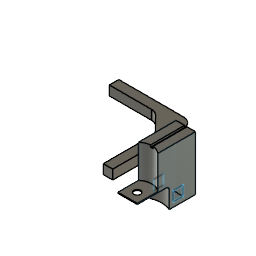
motor_holder_2 (Autodesk Fusion 360 design; units mm, degrees)
part number: 2025-11-13-17-57-27-418
part number: 2025-11-14-11-12-25-876
part number: 2025-11-14-11-12-42-976
Autodesk Fusion 360 part; units mm, degrees
sketch "Sketch1" plane through (0, 0, 0) normal (0, 0, 1) x (1, 0, 0)
  line L0 (0, 0) -> (100, 0)
  line L1 (100, 0) -> (100, 30)
  line L2 (100, 30) -> (0, 30)
  line L3 (0, 30) -> (0, 0)
  line L4 (20, 30) -> (80, 30)
  line L5 (80, 30) -> (80, 0)
  line L6 (80, 0) -> (20, 0)
  line L7 (20, 0) -> (20, 30)
  dimension "d1" = 100
  dimension "d2" = 30
  dimension "d3" = 60
  constraint horizontal L0
  constraint vertical L1
  constraint horizontal L2
  constraint vertical L3
  constraint coincident L0.start L3.end
  constraint horizontal L4
  constraint vertical L5
  constraint horizontal L6
  constraint vertical L7
  constraint coincident L0 L5.end
  constraint coincident L2 L4.start
  constraint midpoint L2 L4
  measures "d1" distance of L0.start L0.end
  measures "d2" distance of L0.start L2.end
  measures "d3" distance of L5 L7
extrude "Extrude2" add sketch "Sketch1" along normal blind 56 contours L0 L2 L3 L7 makes body 1
sketch "Sketch2" plane through (0, 0, 0) normal (0, -1, 0) x (1, 0, 0)
  line L0 (0, 0) -> (20, 0)
  line L1 (20, 0) -> (20, 56)
  line L2 (20, 56) -> (0, 56)
  line L3 (0, 56) -> (0, 0)
  line L4 (0, 56) -> (20, 56)
  line L5 (20, 56) -> (20, 21)
  line L6 (20, 21) -> (0, 21)
  line L7 (0, 21) -> (0, 56)
  line L8 (80, 60) -> (100, 60)
  line L9 (100, 60) -> (100, 30)
  line L10 (100, 30) -> (80, 30)
  line L11 (80, 30) -> (80, 60)
  dimension "d8" = 35
  dimension "d45" = 20
  constraint horizontal L4
  constraint vertical L5
  constraint horizontal L6
  constraint vertical L7
  constraint coincident L2.end L3.start
  constraint horizontal L8
  constraint vertical L9
  constraint horizontal L10
  constraint vertical L11
  measures "d8" distance of L2.end L6.end
  measures "d45" distance of L5 L7
extrude "Extrude3" add sketch "Sketch2" along normal blind 30 contours L1 L2 L3 L4 L5 L6 L7 bodies 1
sketch "Sketch3" plane through (0, 0, 21) normal (0, 0, -1) x (1, 0, 0)
  line L0 (20, 0) -> (20, 30)
  line L1 (20, 30) -> (0, 30)
  line L2 (0, 30) -> (0, 0)
  circle A0 centre (10, 20) radius 3.5
  line L3 (0, 0) -> (20, 0)
  dimension "d11" = 7
  dimension "d13" = 10
  dimension "d15" = 10
  measures "d11" diameter of A0
  measures "d13" distance of L1 A0.centre
  measures "d15" distance of L2 A0.centre
sketch "Sketch4" plane through (0, 0, 56) normal (0, 0, 1) x (-1, 0, 0)
  line L0 (-20, 30) -> (-20, -30)
  line L1 (-20, -30) -> (0, -30)
  line L2 (0, -30) -> (0, 30)
  line L3 (0, 30) -> (-20, 30)
  circle A0 centre (-10, 20) radius 15
  circle A1 centre (-90, 20) radius 15
  dimension "d17" = 30
  dimension "d18" = 30
  measures "d17" diameter of A0
  measures "d18" diameter of A1
extrude "Extrude4" cut sketch "Sketch4" against normal blind 34 contours L0 L2 L3 A0 picked at (-10, 21.6667) bodies 1
extrude "Extrude5" cut sketch "Sketch3" against normal blind 2 contours A0 bodies 1
sketch "Sketch6" plane through (0, 0, 21) normal (0, 0, -1) x (1, 0, 0)
  circle A0 centre (10, 20) radius 20
  circle A1 centre (10, 20) radius 25
  circle A2 centre (10, 20) radius 3.5
  line L0 (20, 30) -> (20, 8.8197)
  arc A3 (0, 8.8197) -> (20, 8.8197) centre (10, 20) ccw
  line L1 (0, 8.8197) -> (0, 30)
  line L2 (0, 30) -> (20, 30)
  circle A4 centre (10, 20) radius 3.5
  line L3 (0, 0) -> (20, 0)
  line L4 (20, 0) -> (20, 30)
  line L5 (20, 30) -> (0, 30)
  line L6 (0, 30) -> (0, 0)
  dimension "d27" = 40
  dimension "d28" = 5
  measures "d27" diameter of A0
extrude "Extrude6" cut sketch "Sketch6" along normal blind 25 contours A0 L3 L6 | A0 L3 L4 | A1 bodies 1
fillet "Fillet2" radius 3 1 edges at (10, 5, 21) on bodies 1
sketch "Sketch7" plane through (0, 0, 56) normal (0, 0, 1) x (-1, 0, 0)
  line L0 (-20, 8.8197) -> (-20, -30)
  line L1 (-20, -30) -> (0, -30)
  line L2 (0, -30) -> (0, 8.8197)
  line L3 (-8.75, 5.0522) -> (-11.25, 5.0522)
  line L4 (-11.25, 5.0522) -> (-11.25, -30)
  line L5 (-11.25, -30) -> (-8.75, -30)
  line L6 (-8.75, -30) -> (-8.75, 5.0522)
  line L7 (0, 5.0522) -> (-20, 5.0522) construction
  arc A0 (-20, 8.8197) -> (0, 8.8197) centre (-10, 20) ccw
  dimension "d33" = 2.5
  constraint horizontal L3
  constraint vertical L4
  constraint horizontal L5
  constraint vertical L6
  constraint coincident L1 L4.end
  constraint coincident L2 L7.start
  constraint coincident L0 L7.end
  constraint perpendicular L0 L7
  constraint midpoint L3 L7
  measures "d33" distance of L4 L6
sketch "Sketch8" plane through (0, 0, 0) normal (-1, 0, 0) x (0, -1, 0)
  line L0 (-2.9129, 0) -> (-2.9129, 18)
  spline S0 degree 3 poles (0.4041, 21) (-0.0235, 21) (-0.5283, 20.9083) (-1.2987, 20.607) (-1.7061, 20.3539) (-2.269, 19.8209) (-2.5307, 19.454) (-2.8238, 18.7805) (-2.9129, 18.359) (-2.9129, 18) knots 1.421755 1.421755 1.421755 1.421755 1.550024 1.550024 1.669923 1.669923 1.782589 1.782589 1.890287 1.890287 1.890287 1.890287
  line L1 (0.4041, 21) -> (30, 21)
  line L2 (30, 21) -> (30, 22)
  line L3 (30, 22) -> (8.8197, 22)
  line L4 (8.8197, 22) -> (8.8197, 56)
  line L5 (8.8197, 56) -> (-30, 56)
  line L6 (-30, 56) -> (-30, 0)
  line L7 (-30, 0) -> (-2.9129, 0)
  line L8 (-17, 15) -> (-7, 15)
  line L9 (-7, 15) -> (-7, 5)
  line L10 (-7, 5) -> (-17, 5)
  line L11 (-17, 5) -> (-17, 15)
  dimension "d37" = 10
  dimension "d38" = 5
  constraint horizontal L8
  constraint vertical L9
  constraint horizontal L10
  constraint vertical L11
  measures "d37" distance of L8.start L10.end
  measures "d38" distance of L7 L10
extrude "Extrude7" cut sketch "Sketch8" against normal blind 9 contours L8 L9 L10 L11 bodies 1
sketch "Sketch9" plane through (20, 0, 0) normal (1, 0, 0) x (0, 1, 0)
  line L0 (2.9129, 0) -> (30, 0)
  line L1 (30, 0) -> (30, 56)
  line L2 (30, 56) -> (-8.8197, 56)
  line L3 (-8.8197, 56) -> (-8.8197, 22)
  line L4 (-8.8197, 22) -> (-30, 22)
  line L5 (-30, 22) -> (-30, 21)
  line L6 (-30, 21) -> (-0.4041, 21)
  spline S0 degree 3 poles (2.9129, 18) (2.9129, 18.359) (2.8238, 18.7805) (2.5307, 19.454) (2.269, 19.8209) (1.7061, 20.3539) (1.2987, 20.607) (0.5283, 20.9083) (0.0235, 21) (-0.4041, 21) knots 0 0 0 0 0.107698 0.107698 0.220364 0.220364 0.340263 0.340263 0.468532 0.468532 0.468532 0.468532
  line L7 (2.9129, 18) -> (2.9129, 0)
  line L8 (7, 15) -> (17, 15)
  line L9 (17, 15) -> (17, 5)
  line L10 (17, 5) -> (7, 5)
  line L11 (7, 5) -> (7, 15)
  constraint horizontal L8
  constraint vertical L9
  constraint horizontal L10
  constraint vertical L11
extrude "Extrude8" cut sketch "Sketch9" against normal blind 9 contours L8 L9 L10 L11 bodies 1
extrude "Extrude9" cut sketch "Sketch7" against normal blind 2 contours L1 L4 L5 L6 A0 bodies 1
sketch "Sketch14" plane through (0, 0, 0) normal (0, 1, 0) x (1, 0, 0)
  line L0 (-45, -10) -> (-35.2, -10)
  line L1 (-35.2, -10) -> (-35.2, -0.2)
  line L2 (-35.2, -0.2) -> (-45, -0.2)
  line L3 (-45, -0.2) -> (-45, -10)
  dimension "d69" = 9.8
  dimension "d70" = 9.8
  constraint horizontal L0
  constraint vertical L1
  constraint horizontal L2
  constraint vertical L3
  measures "d69" distance of L0.start L0.end
  measures "d70" distance of L0.start L2.end
extrude "Extrude15" add sketch "Sketch14" along normal blind 83 separate body makes body 2
sketch "Sketch15" plane through (-45, 0, 0) normal (-1, 0, 0) x (0, -1, 0)
  line L0 (0, 0.2) -> (0, 10)
  line L1 (0, 10) -> (-83, 10)
  line L2 (-83, 10) -> (-83, 0.2)
  line L3 (-83, 0.2) -> (0, 0.2)
  line L4 (-83, 10) -> (-73.2, 10)
  line L5 (-73.2, 10) -> (-73.2, 0.2)
  line L6 (-73.2, 0.2) -> (-83, 0.2)
  line L7 (-83, 0.2) -> (-83, 10)
  dimension "d60" = 9.8
  dimension "d72" = 9.8
  constraint horizontal L4
  constraint vertical L5
  constraint horizontal L6
  constraint vertical L7
  constraint coincident L1.end L2.start
  measures "d60" distance of L1.end L4.end
  measures "d72" distance of L4 L6
extrude "Extrude16" add sketch "Sketch15" along normal blind 67 contours L1 L2 L3 L4 L5 L6 L7 bodies 2
copy_body "Body->Comp1" bodies 2 removing the originals makes body 3 in component "dubel"
copy_body "Body->Comp2" bodies 1 removing the originals makes body 4 in component "motor_holder"
sketch "Sketch16" plane through (0, 0, 10) normal (0, 0, 1) x (-1, 0, 0)
  line L0 (45, 0) -> (35.2, 0)
  line L1 (35.2, 0) -> (35.2, -83)
  line L2 (35.2, -83) -> (112, -83)
  line L3 (112, -83) -> (112, -73.2)
  line L4 (112, -73.2) -> (45, -73.2)
  line L5 (45, -73.2) -> (45, 0)
  line L6 (64.3141, -73.2) -> (45, -73.2)
  line L7 (45, -53.5452) -> (64.3141, -73.2)
  constraint coincident L4 L6.start
  constraint coincident L4.end L5.start
  constraint coincident L5 L7.start
extrude "Extrude1" add sketch "Sketch16" against normal up to surface (9.8 mm away) contours L4 L5 L6 L7 bodies 3 in component "dubel"
fillet "Fillet1" radius 10 2 edges at (-64.3141, 73.2, 5.1) (-45, 53.5452, 5.1) on bodies 3 in component "dubel"
fillet "Fillet2'" radius 10 1 edges at (-35.2, 83, 5.1) on bodies 3 in component "dubel"
component "dubel" placed x (1, 0, 0) y (0, 1, 0) z (0, 0, 1) at (0, 0, 0)
component "motor_holder" placed x (1, 0, 0) y (0, 1, 0) z (0, 0, 1) at (0, 0, 0)
